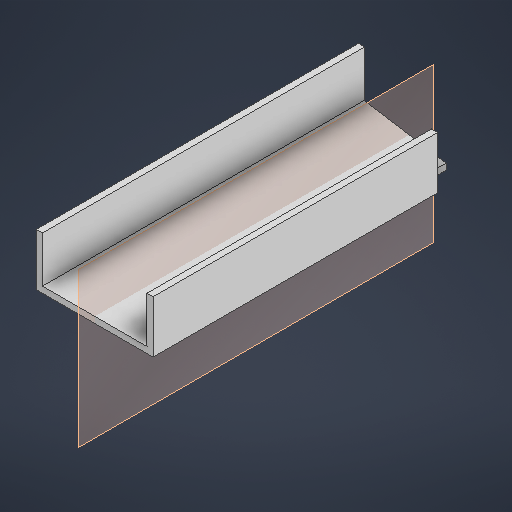
# Autodesk Inventor part: outslideleft
Saved by Autodesk Inventor 2026.2 (Build 302298000, 298)
## iProperties
Created: 2026-02-23
Part Number: outslideleft
Material: Generic
Document SubType Name: Sheet Metal
Designer: danda
Density: 1 g/cm^3
Sheet Metal Rule: Default_mm
Appearance: Default
Author: danda
Autodesk Inventor part; units mm, degrees
ref_plane "XZ Plane" through (0, 0, 0) normal (0, 1, 0) x (-1, 0, 0)
ref_plane "XY Plane" through (0, 0, 0) normal (0, 0, 1) x (1, 0, 0)
sketch "Sketch1" plane through (0, 0, 0) normal (0, 0, 1) x (1, 0, 0)
  line L0 (10.7104, 9.7791) -> (42.7104, 9.7791)
  line L1 (42.7104, 9.7791) -> (42.7104, 24.7791)
  line L2 (10.7104, 9.7791) -> (10.7104, 24.7791)
  line L3 (8.7104, 24.7791) -> (8.7104, 7.7791)
  line L4 (8.7104, 7.7791) -> (44.7104, 7.7791)
  line L5 (44.7104, 7.7791) -> (44.7104, 24.7791)
  line L6 (8.7104, 24.7791) -> (10.7104, 24.7791)
  line L7 (42.7104, 24.7791) -> (44.7104, 24.7791)
  point P0 (0, 0)
  dimension "d0" = 32
  dimension "d1" = 15
  dimension "d2" = 15
  dimension "d3" = 2
  constraints: 16 end point, 3 horizontal, 2 perpendicular, 1 vertical, 2 other
  measures "d0" distance of L0.start L0.end
  measures "d1" distance of L0.end L1.end
  measures "d2" distance of L0.start L2.end
  measures "d3" distance between parallel lines of L2 L3
extrude "Extrusion1" add sketch "Sketch1" along normal blind 100 and the other way blind 5
sketch "Sketch3" plane through (10.7104, 9.7791, 100) normal (0, 1, 0) x (1, 0, 0)
  line L0 (-2, 105) -> (-2, 0) projected
  line L1 (-2, 91.8971) -> (-2, 105)
  line L2 (32, 105) -> (34, 105) projected
  line L3 (34, 105) -> (-2, 91.8971)
  line L4 (-2, 105) -> (-2, 91.8971)
  line L5 (-2, 105) -> (34, 105)
  line L6 (0, 105) -> (0, 0) projected
  line L7 (0, 92.625) -> (0, 105)
  line L8 (34, 105) -> (-2, 99.9405)
  line L9 (34, 105) -> (70.3538, 105) construction
  line L10 (-2, 99.9405) -> (-2, 105)
  point P0 (-10.7104, 100)
  point P1 (-2, 99.9405)
  point P2 (0, 100.2216)
  dimension "d15" = 20
  dimension "d16" = 172
  constraints: 16 end point, 4 point on line, 3 collinear, 1 equal length, 1 horizontal, 1 perpendicular
  measures "d15" angle of L3 L5
  measures "d16" angle of L8 L9
extrude "Extrusion4" cut sketch "Sketch3" along normal through all both and the other way through all contours L5 L6 L8 L0 | L5 L2 L8 L6
extrude "Extrusion5" cut sketch "Sketch3" along normal through all both and the other way through all contours L8 L6 L3 L0
ref_plane "Work Plane1" through (25.71, 0, 0) normal (1, 0, 0) x (0, 1, 0)
mirror "Mirror1" about plane through (25.71, 0, 0) normal (1, 0, 0) of "Extrusion5", "Extrusion4", "Extrusion1"
sketch "Sketch4" plane through (44.7104, 7.7791, 100) normal (1, 0, 0) x (0, 0, -1)
  line L0 (92.625, 2) -> (92.625, 17) projected
  line L1 (92.625, 17) -> (92.625, 2)
  line L2 (92.625, 2) -> (105, 2)
  line L3 (105, 17) -> (105, 0) projected
  line L4 (104.7189, 17) -> (0, 17) projected
  line L5 (105, 17) -> (93.3527, 17)
  line L6 (92.625, 2) -> (92.625, 0)
  line L7 (105, 0) -> (0, 0) projected
  line L8 (92.625, 0) -> (105, 0)
  line L9 (105, 0) -> (105, 2)
  line L10 (92.625, 17) -> (0, 17)
  line L11 (0, 0) -> (0, 17) projected
  line L12 (91.8971, 2) -> (0, 2) projected
  line L13 (0, 2) -> (91.8971, 2)
  point P0 (100, -7.7791)
  point P1 (95.3874, 17)
  constraints: 16 end point, 5 collinear, 2 point on line, 2 vertical, 1 perpendicular
sketch "Sketch5" plane through (25.71, 0, 0) normal (1, 0, 0) x (0, 1, 0)
  line L0 (7.7791, 100) -> (24.7791, 100) projected
  line L1 (24.7791, 100) -> (9.7791, 100)
  line L2 (7.7791, 7.375) -> (9.7791, 7.375) projected
  line L3 (9.7791, 100) -> (9.7791, 7.375)
  line L4 (9.7791, 7.375) -> (24.7791, 7.375)
  line L5 (24.7791, 7.375) -> (24.7791, 100)
  line L6 (9.7791, 7.375) -> (9.7791, 100)
  point P0 (0, 0)
  dimension "d24" = 15
  constraints: 10 end point, 2 perpendicular, 1 collinear, 1 point on line
  measures "d24" distance of L0.end L1.end
extrude "Extrusion7" cut sketch "Sketch5" along normal mid plane 34
extrude "Extrusion8" cut sketch "Sketch4" against normal blind 5 contours L0 L4 L5 L3 L2 | L2 L3 L7 L6
equation "\"BendRadius\" = Thickness"
equation "\"BendReliefWidth\" = Thickness"
equation "\"BendReliefDepth\" = 0.5 * Thickness"
equation "\"CornerReliefSize\" = 4 * Thickness"
equation "\"MinimumRemnant\" = 2 * Thickness"
equation "\"TransitionRadius\" = BendRadius"
equation "\"JacobiRadiusSize\" = BendRadius"
equation "\"GapSize\" = Thickness"
equation "\"Thickness\" = 0.5"
body "Solid1"
